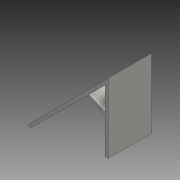
# Autodesk Inventor part: 45度角件
Saved by Autodesk Inventor 2016 (Build 200138000, 138)
## iProperties
Created: 2019-05-19
Part Number: 45度角件
Material: 常规
Document SubType Name: Modeling
Designer: oldboy
Density: 1 g/cm^3
Appearance: 默认
Author: oldboy
Autodesk Inventor part; units mm, degrees
ref_plane "YZ Plane" through (0, 0, 0) normal (1, 0, 0) x (0, 1, 0)
ref_plane "XZ Plane" through (0, 0, 0) normal (0, 1, 0) x (-1, 0, 0)
ref_plane "XY Plane" through (0, 0, 0) normal (0, 0, 1) x (1, 0, 0)
sketch "草图1" plane through (0, 0, 0) normal (0, 1, 0) x (-1, 0, 0)
  line L0 (3, -60) -> (0, -60)
  line L1 (0, -60) -> (0, 0)
  line L2 (45.4264, -42.4264) -> (47.5477, -40.3051)
  line L3 (47.5477, -40.3051) -> (0, 7.2426)
  line L4 (0, 0) -> (0, 7.2426)
  line L5 (3, -22.3594) -> (18.8105, -15.8105)
  line L6 (21.1066, -18.1066) -> (3, -25.6066)
  line L7 (3, 0) -> (18.8105, -15.8105)
  line L8 (21.1066, -18.1066) -> (45.4264, -42.4264)
  line L9 (3, 0) -> (3, -22.3594)
  line L10 (3, -25.6066) -> (3, -60)
  dimension "d3" = 60
  dimension "d6" = 3
  constraints: 22 end point, 3 parallel, 1 perpendicular, 1 vertical
  measures "d3" distance of L7.start L2.start
  measures "d6" distance between parallel lines of L6 L5
extrude "拉伸1" add sketch "草图1" along normal blind 42
sketch "草图2" plane through (-47.5477, 0, -40.3051) normal (-0.7071068, 0, -0.7071068) x (-0.7071068, 0, 0.7071068)
  line L0 (-3, 0) -> (0, 0) projected
  line L1 (0, 0) -> (0, 42) projected
  line L2 (-3, 42) -> (0, 42) projected
  line L3 (-3, 0) -> (-3, 42) projected
  point P0 (-5.1213, 0)
extrude "拉伸2" add sketch "草图2" along normal blind 42
sketch "草图3" plane through (-21.1066, 0, -18.1066) normal (0.7071068, 0, -0.7071068) x (-0.7071068, 0, -0.7071068)
  line L0 (0, 0) -> (76.3934, 0) projected
  line L1 (76.3934, 42) -> (76.3934, 0) projected
  line L2 (0, 42) -> (76.3934, 42) projected
  line L3 (0, 0) -> (0, 42) projected
  circle A0 centre (55.3934, 21) radius 15
  point P0 (-27.7279, 0)
  dimension "d11" = 30
  dimension "d12" = 21
  dimension "d13" = 21
  constraints: 1 centre point
  measures "d11" diameter of A0
  measures "d12" distance from line of L0 A0.centre
  measures "d13" distance from line of L1 A0.centre
extrude "拉伸3" cut sketch "草图3" against normal blind 42 contours A0
